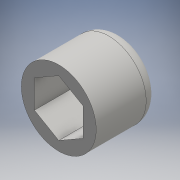
# Autodesk Inventor part: Nut
Saved by Autodesk Inventor 2016 (Build 200138000, 138)
## iProperties
Created: 2016-12-05
Part Number: Nut
Material: Generic
Document SubType Name: Modeling
Designer: Muhammad
Density: 1 g/cm^3
Appearance: Default
Author: Muhammad
Autodesk Inventor part; units mm, degrees
ref_plane "YZ Plane" through (0, 0, 0) normal (1, 0, 0) x (0, 1, 0)
ref_plane "XZ Plane" through (0, 0, 0) normal (0, 1, 0) x (-1, 0, 0)
ref_plane "XY Plane" through (0, 0, 0) normal (0, 0, 1) x (1, 0, 0)
sketch "Sketch1" plane through (0, 0, 0) normal (0, 1, 0) x (-1, 0, 0)
  circle A0 centre (0, 0) radius 2.25
  circle A1 centre (0, 0) radius 3
  dimension "d0" = 4.5
  dimension "d1" = 6
  constraints: 2 centre point, 2 coincident
  measures "d0" diameter of A0
  measures "d1" diameter of A1
extrude "Extrusion1" add sketch "Sketch1" along normal blind 5 contours A0 | A1
sketch "Sketch2" plane through (0, 5, 0) normal (0, 1, 0) x (1, 0, 0)
  line L0 (0, 0) -> (0, 2.25)
  line L1 (0, 2.25) -> (1.9486, 1.125)
  line L2 (1.9486, 1.125) -> (1.9486, -1.125)
  line L3 (1.9486, -1.125) -> (0, -2.25)
  line L4 (0, -2.25) -> (-1.9486, -1.125)
  line L5 (-1.9486, -1.125) -> (-1.9486, 1.125)
  line L6 (-1.9486, 1.125) -> (0, 2.25)
  dimension "d4" = 2.25
  constraints: 14 end point, 1 coincident, 1 vertical, 13 other
  measures "d4" distance of L0.start L0.end
extrude "Extrusion2" cut sketch "Sketch2" against normal through all
fillet "Fillet1" radius 1 1 edges at (3, 5, 0)
body "Solid1"
